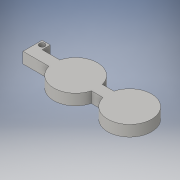
# Autodesk Inventor part: wheels
Saved by Autodesk Inventor 2016 (Build 200138000, 138)
## iProperties
Created: 2018-01-19
Part Number: wheels
Material: Generic
Document SubType Name: Modeling
Designer: New User
Density: 1 g/cm^3
Appearance: Default
Author: New User
Autodesk Inventor part; units mm, degrees
ref_plane "YZ Plane" through (0, 0, 0) normal (1, 0, 0) x (0, 1, 0)
ref_plane "XZ Plane" through (0, 0, 0) normal (0, 1, 0) x (-1, 0, 0)
ref_plane "XY Plane" through (0, 0, 0) normal (0, 0, 1) x (1, 0, 0)
sketch "Sketch1" plane through (0, 0, 0) normal (0, 1, 0) x (-1, 0, 0)
  line L0 (0, 0) -> (19.05, 0)
  line L1 (19.05, 0) -> (19.05, 44.45)
  line L2 (0, 19.05) -> (0, 0)
  circle A0 centre (9.525, 9.525) radius 6.35
  arc A1 (-166.7131, 44.45) -> (-166.7131, 19.05) centre (-215.9, 31.75) ccw
  line L3 (19.05, 44.45) -> (-41.3006, 44.45)
  line L4 (-139.6744, 44.45) -> (-166.7131, 44.45)
  line L5 (-166.7131, 19.05) -> (-139.6744, 19.05)
  line L6 (-41.3006, 19.05) -> (0, 19.05)
  arc A2 (-41.3006, 44.45) -> (-139.6744, 44.45) centre (-90.4875, 31.75) ccw
  arc A3 (-139.6744, 19.05) -> (-41.3006, 19.05) centre (-90.4875, 31.75) ccw
  dimension "d0" = 19.05
  dimension "d2" = 12.7
  dimension "d5" = 44.45
  constraints: 14 end point, 6 point on circle, 4 centre point, 3 perpendicular, 1 horizontal
  measures "d0" distance between parallel lines of L1 L2
  measures "d2" diameter of A0
  measures "d5" distance of L0.end L1.end
extrude "Extrusion1" add sketch "Sketch1" along normal blind 25.4
body "Solid1"
